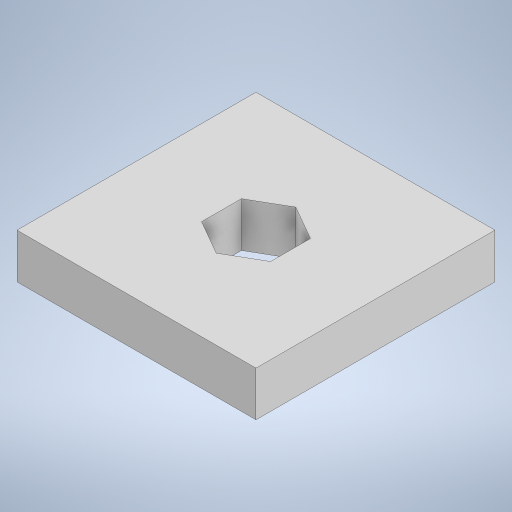
# Autodesk Inventor part: Hex Box
Saved by Autodesk Inventor 2023 (Build 270158000, 158)
## iProperties
Created: 2023-01-21
Part Number: Hex Box
Material: Generic
Document SubType Name: Modeling
Designer: bugme
Density: 1 g/cm^3
Appearance: Default
Author: bugme
Autodesk Inventor part; units mm, degrees
ref_plane "YZ Plane" through (0, 0, 0) normal (1, 0, 0) x (0, 1, 0)
ref_plane "XZ Plane" through (0, 0, 0) normal (0, 1, 0) x (-1, 0, 0)
ref_plane "XY Plane" through (0, 0, 0) normal (0, 0, 1) x (1, 0, 0)
sketch "Sketch1" plane through (0, 0, 0) normal (0, 1, 0) x (-1, 0, 0)
  line L0 (50.8, 0) -> (50.8, 50.8)
  line L1 (50.8, 50.8) -> (0, 50.8)
  line L2 (0, 50.8) -> (0, 0)
  line L3 (0, 0) -> (50.8, 0)
  line L4 (25.4, 16.9333) -> (18.0677, 21.1667)
  line L5 (18.0677, 21.1667) -> (18.0677, 29.6333)
  line L6 (18.0677, 29.6333) -> (25.4, 33.8667)
  line L7 (25.4, 33.8667) -> (32.7323, 29.6333)
  line L8 (32.7323, 29.6333) -> (32.7323, 21.1667)
  line L9 (32.7323, 21.1667) -> (25.4, 16.9333)
  point P0 (25.4, 25.4)
  point P1 (21.7338, 19.05)
  point P2 (29.0662, 31.75)
  dimension "d0" = 50.8
  dimension "d1" = 50.8
  dimension "d4" = 12.7
  constraints: 20 end point, 2 midpoint, 2 perpendicular, 1 parallel, 1 vertical, 13 other
  measures "d0" distance of L0.start L0.end
  measures "d1" distance of L0.end L1.end
  measures "d4" vertical distance of point (21.734, 19.05) point (29.066, 31.75)
extrude "Extrusion1" add sketch "Sketch1" along normal mid plane 9.525
body "Solid1"
